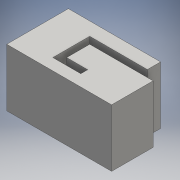
# Autodesk Inventor part: endstop mount
Saved by Autodesk Inventor 2016 SP1 (Build 200210100, 210)
## iProperties
Created: 2017-05-11
Part Number: endstop mount
Material: Generic
Document SubType Name: Modeling
Designer: Cole
Density: 1 g/cm^3
Appearance: Default
Author: Cole
Autodesk Inventor part; units mm, degrees
ref_plane "YZ Plane" through (0, 0, 0) normal (1, 0, 0) x (0, 1, 0)
ref_plane "XZ Plane" through (0, 0, 0) normal (0, 1, 0) x (-1, 0, 0)
ref_plane "XY Plane" through (0, 0, 0) normal (0, 0, 1) x (1, 0, 0)
sketch "Sketch1" plane through (0, 0, 0) normal (0, 0, 1) x (1, 0, 0)
  line L0 (0, 7.7) -> (0, 1.3)
  line L1 (1.2, 6.5) -> (12.2, 6.5)
  line L2 (1.2, 2.5) -> (4.8537, 2.5)
  line L3 (1.2, 6.5) -> (1.2, 2.5)
  line L4 (0, 1.3) -> (4.8537, 1.3)
  line L5 (4.8537, 2.5) -> (4.8537, 1.3)
  line L6 (12.2, -0.7) -> (12.2, 6.5)
  line L7 (0, 7.7) -> (10, 7.7)
  line L8 (10, 7.7) -> (10, 10)
  line L9 (-6, 10) -> (-6, -0.7)
  line L10 (-6, 10) -> (10, 10)
  line L11 (-6, -0.7) -> (12.2, -0.7)
  dimension "d7" = 1.2
  dimension "d9" = 1.2
  dimension "d10" = 11
  dimension "d12" = 1.2
  dimension "d13" = 4
  dimension "d21" = 6
  constraints: 24 end point, 1 horizontal, 1 perpendicular
  measures "d7" distance between parallel lines of L0 L3
  measures "d9" distance between parallel lines of L4 L2
  measures "d10" distance between parallel lines of L6 L3
  measures "d12" distance between parallel lines of L1 L7
  measures "d13" distance between parallel lines of L2 L1
  measures "d21" distance between parallel lines of L9 L0
extrude "Extrusion3" add sketch "Sketch1" along normal blind 10
sketch "Sketch3" plane through (-6, -0.7, 0) normal (-1, 0, 0) x (0, 0, 1)
  circle A0 centre (5, 8.5811) radius 1
  circle A1 centre (5, 2.0811) radius 1
  line L0 (0, 0) -> (0, 10.7) projected
  line L1 (0, 0) -> (10, 0) projected
  line L2 (10, 10.7) -> (10, 0) projected
  line L3 (0, 10.7) -> (10, 10.7) projected
  line L4 (5, 10.7) -> (5, 0)
  point P0 (0, 0.7)
  dimension "d24" = 2
  dimension "d25" = 2
  dimension "d26" = 6.5
  constraints: 2 centre point, 2 end point, 2 point on line
  measures "d24" diameter of A1
  measures "d25" diameter of A0
  measures "d26" distance of A1.centre A0.centre
extrude "Extrusion4" cut sketch "Sketch3" against normal blind 6 contours A0 L4 | L4 A0 | L4 A1 | A1 L4
body "Solid2"
